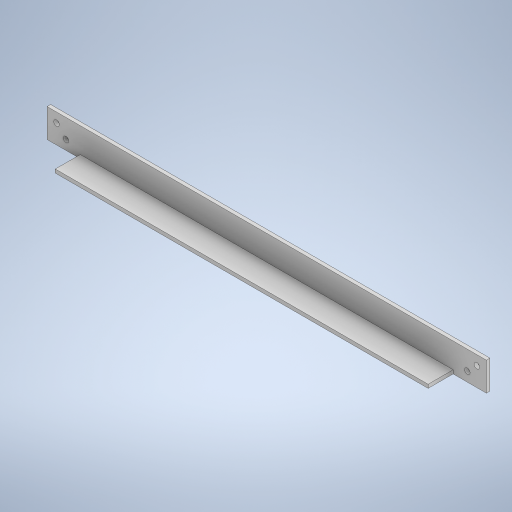
# Autodesk Inventor part: beamZ
Saved by Autodesk Inventor 2023 (Build 270158000, 158)
## iProperties
Created: 2023-06-23
Part Number: beamZ
Material: Generic
Document SubType Name: Modeling
Designer: incep
Density: 1 g/cm^3
Appearance: Default
Author: incep
Autodesk Inventor part; units mm, degrees
ref_plane "YZ Plane" through (0, 0, 0) normal (1, 0, 0) x (0, 1, 0)
ref_plane "XZ Plane" through (0, 0, 0) normal (0, 1, 0) x (-1, 0, 0)
ref_plane "XY Plane" through (0, 0, 0) normal (0, 0, 1) x (1, 0, 0)
sketch "Sketch1" plane through (0, 0, 0) normal (1, 0, 0) x (0, 1, 0)
  line L0 (25.4, 25.4) -> (0, 25.4) construction
  line L1 (0, 25.4) -> (0, 0)
  line L2 (0, 0) -> (25.4, 0)
  line L3 (25.4, 0) -> (25.4, 25.4) construction
  line L4 (25.4, 25.4) -> (3.175, 25.4) construction
  line L5 (3.175, 25.4) -> (3.175, 3.175)
  line L6 (3.175, 3.175) -> (25.4, 3.175)
  line L7 (25.4, 3.175) -> (25.4, 25.4) construction
  line L8 (25.4, 3.175) -> (25.4, 0)
  line L9 (3.175, 25.4) -> (0, 25.4)
  point P0 (0, 0)
  dimension "d1" = 25.4
  dimension "d2" = 3.175
  constraints: 20 end point, 5 perpendicular, 4 parallel, 2 horizontal, 1 coincident, 1 collinear
  measures "d1" distance of L0.start L0.end
  measures "d2" distance between parallel lines of L2 L6
extrude "Extrusion1" add sketch "Sketch1" along normal mid plane 390.8
sketch "Sketch2" plane through (-195.4, 3.175, 25.4) normal (0, 1, 0) x (1, 0, 0)
  line L0 (0, 0) -> (390.8, 0) projected
  line L1 (0, 0) -> (29.575, 0)
  line L2 (29.575, 0) -> (29.575, 22.225)
  line L3 (29.575, 22.225) -> (0, 22.225)
  line L4 (0, 22.225) -> (0, 0)
  line L5 (0, 22.225) -> (390.8, 22.225) projected
  point P0 (195.4, 25.4)
  point P1 (29.575, 0)
  dimension "d5" = 29.575
  constraints: 8 end point, 2 parallel, 1 horizontal, 1 perpendicular, 1 point on line
  measures "d5" distance between parallel lines of L2 L4
extrude "Extrusion2" cut sketch "Sketch2" against normal blind 3.175
sketch "Sketch3" plane through (-195.4, 25.4, 3.175) normal (0, 0, 1) x (1, 0, 0)
  line L0 (0, 0) -> (390.8, 0) construction
  line L1 (0, 0) -> (25.4, 0) construction
  line L2 (25.4, 0) -> (25.4, -25.4) construction
  line L3 (25.4, -25.4) -> (0, -25.4) construction
  line L4 (0, -25.4) -> (0, 0) construction
  line L5 (3.175, 0) -> (22.225, 0) construction
  line L6 (22.225, 0) -> (22.225, -25.4) construction
  line L7 (22.225, -25.4) -> (3.175, -25.4) construction
  line L8 (3.175, -25.4) -> (3.175, 0) construction
  line L9 (8.4667, -8.4667) -> (16.9333, -8.4667) construction
  line L10 (16.9333, -8.4667) -> (16.9333, -16.9333) construction
  line L11 (16.9333, -16.9333) -> (8.4667, -16.9333) construction
  line L12 (8.4667, -16.9333) -> (8.4667, -8.4667) construction
  circle A0 centre (8.4667, -8.4667) radius 2.4257
  circle A1 centre (16.9333, -16.9333) radius 2.4257
  point P0 (195.4, -25.4)
  point P1 (12.7, 0)
  point P2 (12.7, 0)
  point P3 (16.9333, -12.7)
  point P4 (22.225, -12.7)
  point P5 (12.7, -8.4667)
  dimension "d8" = 25.4
  dimension "d9" = 3.175
  dimension "d10" = 4.8514
  dimension "d11" = 8.4667
  constraints: 24 end point, 6 parallel, 5 midpoint, 5 perpendicular, 3 coincident, 3 horizontal, 2 centre point, 2 collinear, 1 equal radius, 1 horizontal alignment, 1 vertical alignment
  measures "d8" distance of L2.end L3.end
  measures "d9" distance between parallel lines of L4 L8
  measures "d10" diameter of A0
  measures "d11" distance of L9.start L9.end
extrude "Extrusion3" cut sketch "Sketch3" against normal blind 3.175
mirror "Mirror1" about plane through (0, 0, 0) normal (1, 0, 0) of "Extrusion2", "Extrusion3"
body "Solid1"
